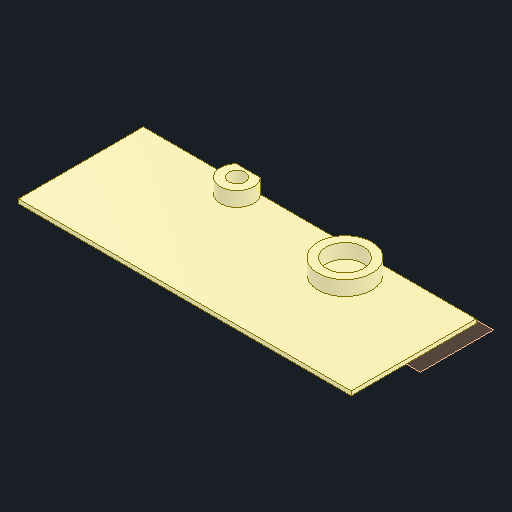
# Autodesk Inventor part: right_gear_holder
Saved by Autodesk Inventor 2023 (Build 270158000, 158)
## iProperties
Created: 2024-05-18
Part Number: right_gear_holder
Material: Nylon 6/6
Document SubType Name: Modeling
Designer: szymo
Density: 1.13 g/cm^3
Appearance: Nylon 6
Mass: 3.11361 g
Surface Area: 53.9129 cm^2
Volume: 2.75541 cm^3
Author: szymo
Autodesk Inventor part; units mm, degrees
ref_plane "YZ Plane" through (0, 0, 0) normal (1, 0, 0) x (0, 1, 0)
ref_plane "XZ Plane" through (0, 0, 0) normal (0, 1, 0) x (-1, 0, 0)
ref_plane "XY Plane" through (0, 0, 0) normal (0, 0, 1) x (1, 0, 0)
ref_plane "Work Plane1" through (23, 8.5, 16) normal (0, 1, 0) x (0, 0, -1)
sketch "Sketch2" plane through (23, 8.5, 16) normal (0, 1, 0) x (0, 0, -1)
  circle A0 centre (1, -3) radius 15 projected
  line L0 (19.5, 94) -> (19.5, -18) projected
  line L1 (16, 94) -> (16, -18) projected
  line L2 (19.5, 94) -> (16, 94) projected
  line L3 (19.5, -18) -> (19.5, -68) projected
  line L4 (19.5, -68) -> (16, -68) projected
  line L5 (16, -18) -> (16, -68) projected
  line L6 (16, 12) -> (-14, 12)
  line L7 (-14, 12) -> (-14, -68)
  line L8 (-14, -68) -> (16, -68)
  line L9 (16, -68) -> (16, 12)
  circle A1 centre (9.5, -43) radius 22.5 projected
  point P0 (16, 23)
  constraints: 8 end point, 2 parallel, 2 tangent, 1 collinear, 1 horizontal, 1 perpendicular, 1 point on line
extrude "Extrusion1" add sketch "Sketch2" along normal blind 1 contours A0 | L1 L5 A1 L8 L7 A0 | A0 L6 L1 | A0 L7 L6 | L5 A1
sketch "Sketch3" plane through (23, 9.5, 16) normal (0, 1, 0) x (1, 0, 0)
  circle A0 centre (43, 9.5) radius 4.5 projected
  circle A1 centre (43, 9.5) radius 2.5 projected
  line L0 (68, -14) -> (68, 16) projected
  line L1 (-12, -14) -> (68, -14) projected
  line L2 (-12, 16) -> (-12, -14) projected
  line L3 (68, 16) -> (-12, 16) projected
  circle A2 centre (13.2408, 13.2933) radius 2 projected
  circle A3 centre (43, 9.5) radius 6.5
  circle A4 centre (13.2408, 13.2933) radius 4
  point P0 (-23, 16)
  point P1 (10.2956, 16)
  point P2 (16.186, 16)
  dimension "d2" = 2
  dimension "d3" = 2
  constraints: 2 centre point
  measures "d2" radial gap between concentric circles of A0 A3
  measures "d3" radial gap between concentric circles of A2 A4
ref_plane "Work Plane2" through (59.7138, 13, 0.2138) normal (0, 1, 0) x (0.588283, 0, 0.8086551)
extrude "Extrusion2" add sketch "Sketch3" along normal up to surface (3.5 mm away) contours A3 | A4 L3 picked at (13.3212, 15.7596)
body "Solid1"
